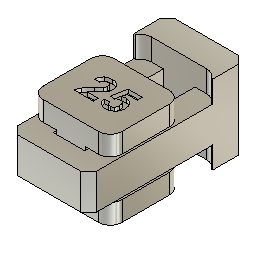
19운용기능사예제1 v1 (Autodesk Fusion 360 design; units mm, degrees)
Autodesk Fusion 360 part; units mm, degrees
sketch "Sketch1" plane through (0, 0, 0) normal (0, 1, 0) x (1, 0, 0)
  line L0 (0, 0) -> (0, 35)
  line L1 (-10, 0) -> (10, 0)
  line L2 (10, 0) -> (10, -5)
  line L3 (10, -5) -> (-10, -5)
  line L4 (-10, -5) -> (-10, 0)
  line L5 (-3.7, -5) -> (3.7, -5)
  line L6 (3.7, -5) -> (3.7, -15)
  line L7 (3.7, -15) -> (-3.7, -15)
  line L8 (-3.7, -15) -> (-3.7, -5)
  line L9 (-10, -15) -> (10, -15)
  line L10 (10, -15) -> (10, -20)
  line L11 (10, -20) -> (-10, -20)
  line L12 (-10, -20) -> (-10, -15)
  dimension "d1" = 20
  dimension "d2" = 20
  dimension "d3" = 7.4
  dimension "d4" = 5
  dimension "d5" = 10
  dimension "d6" = 5
  constraint coincident L0.start origin
  constraint vertical L0
  constraint horizontal L1
  constraint vertical L2
  constraint horizontal L3
  constraint vertical L4
  constraint horizontal L5
  constraint vertical L6
  constraint horizontal L7
  constraint vertical L8
  constraint coincident L3 L5.start
  constraint horizontal L9
  constraint vertical L10
  constraint horizontal L11
  constraint vertical L12
  constraint symmetric L0 L2 L4
  constraint symmetric L0 L6 L8
  constraint symmetric L0 L10 L12
  constraint coincident L6.end L9
  measures "d1" distance of L10.end L11.end
  measures "d2" distance of L1.start L1.end
  measures "d3" distance of L6 L8
  measures "d4" distance of L1.end L2.end
  measures "d5" distance of L5.end L6.end
  measures "d6" distance of L9.end L10.end
extrude "Extrude1" add sketch "Sketch1" along normal blind 18 makes body 1
fillet "Fillet1" radius 3 8 edges at (10, 0, 17.5) (-10, 0, 17.5) (-10, 0, 2.5) (10, 0, 2.5) (10, 18, 17.5) (10, 18, 2.5) (-10, 18, 17.5) (-10, 18, 2.5) on bodies 1
sketch "Sketch2" plane through (0, 0, 20) normal (0, 0, 1) x (-1, 0, 0)
  line L0 (5.1855, -5.8637) -> (-5.3858, -5.8637) construction
  line L1 (-5.3858, -5.8637) -> (-5.3858, -15.8637) construction
  line L2 (-5.3858, -15.8637) -> (5.1855, -15.8637) construction
  line L3 (5.1855, -15.8637) -> (5.1855, -5.8637) construction
  text T0 "25" font "Arial" height 10 bold align ink ink in box 0 x 0 at (5.1755, -5.8837) x (-1, 0) y (0, -1) spacing 1 height is em
  constraint perpendicular L0 L1
  constraint parallel L0 L2
  constraint parallel L1 L3
extrude "Extrude2" cut sketch "Sketch2" against normal blind 1 text T0 bodies 1
sketch "Sketch3" plane through (0, 0, 5) normal (0, 0, 1) x (-1, 0, 0)
  arc A0 (-10, -15) -> (-7, -18) centre (-7, -15) ccw
  line L0 (-7, -18) -> (-3.7, -18)
  line L1 (-3.7, -18) -> (-3.7, 0)
  line L2 (-3.7, 0) -> (-7, 0)
  arc A1 (-7, 0) -> (-10, -3) centre (-7, -3) ccw
  line L3 (-10, -3) -> (-10, -15)
  line L4 (0, 0) -> (0, 1.5)
  line L5 (4, -27.5) -> (-4, -27.5)
  line L6 (-4, -27.5) -> (-4, 0.5)
  line L7 (-4, 0.5) -> (4, 0.5)
  line L8 (4, 0.5) -> (4, -27.5)
  line L9 (10, -34.5) -> (-10, -34.5)
  line L10 (-10, -34.5) -> (-10, 5.5)
  line L11 (-10, 5.5) -> (10, 5.5)
  line L12 (10, 5.5) -> (10, -34.5)
  dimension "d13" = 8
  dimension "d14" = 28
  dimension "d15" = 0.5
  dimension "d16" = 5
  dimension "d34" = 7
  constraint coincident L4.start origin
  constraint vertical L4
  constraint horizontal L5
  constraint vertical L6
  constraint horizontal L7
  constraint vertical L8
  constraint symmetric L4 L6 L8
  constraint horizontal L9
  constraint vertical L10
  constraint horizontal L11
  constraint vertical L12
  constraint symmetric L4 L10 L12
  measures "d13" distance of L6.end L7.end
  measures "d14" distance of L5.end L6.end
  measures "d15" distance of L4.start L7
  measures "d16" distance of L7 L11
  measures "d34" distance of L5 L9
extrude "Extrude3" add sketch "Sketch3" along normal blind 9 from surface at 0.5 separate body contours A0 L0 L2 A1 L3 L6 L10 | A0 L0 L2 A1 L5 L6 L7 L8 L9 L10 L11 L12 makes body 2
sketch "Sketch4" plane through (0, 0, 14.5) normal (0, 0, 1) x (-1, 0, 0)
  line L0 (-4, 0.5) -> (4, 0.5)
  line L1 (4, 0.5) -> (4, -27.5)
  line L2 (4, -27.5) -> (-4, -27.5)
  line L3 (-4, -27.5) -> (-4, 0.5)
  line L4 (10, 5.5) -> (-10, 5.5)
  line L5 (-10, -34.5) -> (10, -34.5)
  line L6 (10, -34.5) -> (10, 5.5)
  line L7 (0, -34.5) -> (0, -39.4337)
  line L8 (10, -27.5) -> (-10, -27.5)
  line L9 (-10, -34.5) -> (10, -34.5)
  circle A0 centre (7, -24.5) radius 3
  circle A1 centre (-7, -24.5) radius 3
  line L10 (13.7534, -26) -> (-13.9932, -26)
  line L11 (10, -34.5) -> (10, -26)
  line L12 (-10, -34.5) -> (-10, -25.5)
  dimension "d20" = 6
  dimension "d21" = 7
  dimension "d22" = 3
  dimension "d23" = 6
  dimension "d24" = 3
  dimension "d25" = 7
  dimension "d27" = 1.5
  constraint midpoint L5 L7.start
  constraint perpendicular L5 L7
  constraint coincident L6 L8.start
  constraint coincident L5.start L9.start
  constraint coincident L5.end L6.start
  constraint collinear L2 L8
  constraint coincident L10 L11.end
  constraint coincident L6 L11.end
  constraint perpendicular L9 L12
  measures "d20" diameter of A0
  measures "d21" distance of L7 A0.centre
  measures "d22" distance of L8 A0.centre
  measures "d23" diameter of A1
  measures "d24" distance of L8 A1.centre
  measures "d25" distance of L7 A1.centre
  measures "d27" distance of L8 L10
extrude "Extrude4" add sketch "Sketch4" along normal blind 5.5 contours L8 A1 L10 L12 | L2 L5 L6 L8 L9 L11 L12 | L6 L8 A0 L10 L11 bodies 2
extrude "Extrude5" add sketch "Sketch4" against normal blind 5.5 from surface at -9 contours L8 A1 L10 L12 | L2 L5 L6 L8 L9 L11 L12 | L6 L8 A0 L10 L11 bodies 2
chamfer "Chamfer1" distance 2 angle 45 4 edges at (-10, -5.5, 10) (10, -5.5, 10) (10, 34.5, 10) (-10, 34.5, 10) on bodies 2
copy_body "Body->Comp1" bodies 1 removing the originals makes body 3 in component "Component'"
copy_body "Body->Comp2" bodies 2 removing the originals makes body 4 in component "Component''"
component "Component'" placed x (1, 0, 0) y (0, 1, 0) z (0, 0, 1) at (0, 0, 0)
component "Component''" placed x (1, 0, 0) y (0, 1, 0) z (0, 0, 1) at (0, 0, 0)
